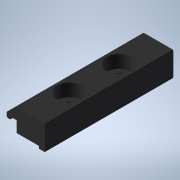
# Autodesk Inventor part: 722624 MUE-70/80P1
Saved by Autodesk Inventor 2021 (Build 250183000, 183)
## iProperties
Created: 2026-04-18
Part Number: 722624 MUE-70/80P1
Material: Generic
Catalog Web Link: www.3dfindit.com
Description: MUE-P1-terminal strip
Vendor: FESTO
Document SubType Name: Modeling
Designer: psAdmin
Manufacturer: FESTO
Mass: 5.20588 g
Surface Area: 32.0188 cm^2
Volume: 5.20588 cm^3
Density: 1 g/cm^3
Appearance: PSOLRGB-176-176-176
Category: PARTsolutions
Company: FESTO
Title: 722624 MUE-70/80P1
Author: Cadenas PARTsolutions
Comments: terminal strip
PSOL_IDENT_0: {$CADENAS_DATA/23d-libs/festo/parts/m/mue/parts/mue_1.prj},176 {VTYP=3D},{NB=722624 MUE-70/80P1},{LI
PSOL_IDENT_1: NA=722624 MUE-70/80P1},{NN=MUE-P1},{DATE=30.06.2025 07:27:24},{GEOMDATE=03.09.2015 14:16:08},{VERSIO
PSOL_IDENT_2: N=},{LINEID=20},{WBVAR=},{WBNUMERIC=}  {NB=722624 MUE-70/80P1},{LINA=722624 MUE-70/80P1},{KT=DUMMY},
PSOL_IDENT_3: {TNR=722624},{TYP=MUE-70/80},{V=3},{B=-0.250},{B1=4.800},{B2=10.000}
NB: 722624 MUE-70/80P1
NN: MUE-P1
NT: terminal strip
NBSYN: $TNR. $TYP.P1
LINA: 722624 MUE-70/80P1
CATALOG: Festo
TNR: 722624
TYP: MUE-70/80
V: 3
B: -0.25
B1: 4.8
B2: 10
SUPPLIER: FESTO
ARTICLENO: 722624 MUE-70/80P1
BOMINFO: 722624 MUE-70/80P1
CREATOR: CADENAS GmbH
Autodesk Inventor part; units mm, degrees
sketch "Sketch_4" plane through (0, 0, 0) normal (0, 0, 1) x (1, 0, 0)
  line L0 (-9.75, 6.2929) -> (-9.75, 5)
  arc A0 (-9.75, 5) -> (-9.25, 4.5) centre (-9.25, 5) ccw
  line L1 (-9.25, 4.5) -> (-8.45, 4.5)
  arc A1 (-8.45, 4.5) -> (-8.25, 4.7) centre (-8.45, 4.7) ccw
  line L2 (-8.25, 4.7) -> (-8.25, 5.3)
  arc A2 (-8.05, 5.5) -> (-8.25, 5.3) centre (-8.05, 5.3) ccw
  line L3 (-8.05, 5.5) -> (-5.95, 5.5)
  arc A3 (-5.75, 5.3) -> (-5.95, 5.5) centre (-5.95, 5.3) ccw
  line L4 (-5.75, 5.3) -> (-5.75, 1.2)
  arc A4 (-5.75, 1.2) -> (-5.55, 1) centre (-5.55, 1.2) ccw
  line L5 (-5.55, 1) -> (3.05, 1)
  arc A5 (3.25, 0.8) -> (3.05, 1) centre (3.05, 0.8) ccw
  line L6 (3.25, 0.8) -> (3.25, 0.2)
  arc A6 (3.25, 0.2) -> (3.45, 0) centre (3.45, 0.2) ccw
  line L7 (3.45, 0) -> (5.55, 0)
  arc A7 (5.55, 0) -> (5.75, 0.2) centre (5.55, 0.2) ccw
  line L8 (5.75, 0.2) -> (5.75, 9.8)
  arc A8 (5.75, 9.8) -> (5.55, 10) centre (5.55, 9.8) ccw
  line L9 (5.55, 10) -> (-6.0429, 10)
  arc A9 (-6.0429, 10) -> (-6.3964, 9.8536) centre (-6.0429, 9.5) ccw
  line L10 (-6.3964, 9.8536) -> (-9.6036, 6.6464)
  arc A10 (-9.6036, 6.6464) -> (-9.75, 6.2929) centre (-9.25, 6.2929) ccw
  constraints: 22 end point, 22 point on circle, 11 centre point
extrude "Extrusion1" add sketch "Sketch_4" along normal mid plane 52
sketch "Sketch2" plane through (-6.0429, 10, 26) normal (0, 1, 0) x (1, 0, 0)
  point P0 (5.7929, 36)
hole "Hole1" at (-0.25, 10, -10) direction (0, -1, 0) diameter 5.5 depth 10 counterbore diameter 10 counterbore depth 5.2
sketch "Sketch3" plane through (-6.0429, 10, 26) normal (0, 1, 0) x (1, 0, 0)
  point P0 (5.7929, 16)
hole "Hole2" at (-0.25, 10, 10) direction (0, -1, 0) diameter 5.5 depth 10 counterbore diameter 10 counterbore depth 5.2
ref_plane "KLEMMLEISTE_XY" through (-0.25, 0, 0) normal (0, 1, 0) x (1, 0, 0)
ref_plane "KLEMMLEISTE_YZ" through (-0.25, 0, 0) normal (1, 0, 0) x (0, 0, -1)
ref_plane "KLEMMLEISTE_ZX" through (-0.25, 0, 0) normal (0, 0, -1) x (0, 1, 0)
ref_plane "SCHRAUBE_1_XY" through (-0.25, 4.8, -10) normal (0, 1, 0) x (1, 0, 0)
ref_plane "SCHRAUBE_1_YZ" through (-0.25, 4.8, -10) normal (1, 0, 0) x (0, 0, -1)
ref_plane "SCHRAUBE_1_ZX" through (-0.25, 4.8, -10) normal (0, 0, -1) x (0, 1, 0)
ref_plane "SCHRAUBE_2_XY" through (-0.25, 4.8, 10) normal (0, 1, 0) x (1, 0, 0)
ref_plane "SCHRAUBE_2_YZ" through (-0.25, 4.8, 10) normal (1, 0, 0) x (0, 0, -1)
ref_plane "SCHRAUBE_2_ZX" through (-0.25, 4.8, 10) normal (0, 0, -1) x (0, 1, 0)
body "Solid1"
